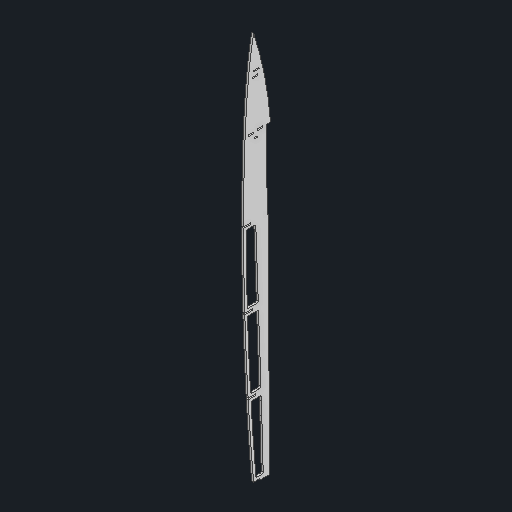
# Autodesk Inventor part: stringer
Saved by Autodesk Inventor 2023 (Build 270158030, 158C)
## iProperties
Created: 2022-03-21
Part Number: stringer
Material: Generic
Document SubType Name: Modeling
Designer: kardo
Density: 1 g/cm^3
Appearance: Default
Mass: 50.8397 g
Surface Area: 402.853 cm^2
Volume: 50.8397 cm^3
Author: kardo
Autodesk Inventor part; units mm, degrees
ref_plane "YZ Plane" through (0, 0, 0) normal (1, 0, 0) x (0, 1, 0)
ref_plane "XZ Plane" through (0, 0, 0) normal (0, 1, 0) x (-1, 0, 0)
ref_plane "XY Plane" through (0, 0, 0) normal (0, 0, 1) x (1, 0, 0)
derived "parameters_frame.ipt"
derived "surface_body.ipt"
sketch "sk_long_outer" plane through (0, 0, 0) normal (1, 0, 0) x (0, 1, 0)
  line L0 (-345, 107.6209) -> (-345, -224.5198) construction
  line L1 (255, 107.6209) -> (255, -224.5198) construction
  line L2 (-465, 54.4) -> (375, 54.4) construction
  line L3 (-483, 0) -> (357, 0) construction
  line L4 (0, 107.6209) -> (0, -224.5198) construction
  line L5 (0, 14.144) -> (-345, 11.968)
  line L6 (-345, 11.968) -> (-345, 39.712)
  line L7 (-345, 39.712) -> (0, 54.4)
  line L8 (0, 54.4) -> (255, 36.448)
  line L9 (0, 0) -> (122.4, 9.6331)
  line L10 (122.4, 9.6331) -> (255, 36.448)
  line L11 (0, 14.144) -> (0, 0)
  line L12 (0, 14.144) -> (121.9006, 15.9783)
  line L13 (121.9006, 15.9783) -> (122.4, 9.6331)
sketch "sk_rail_sponson_tunnel" plane through (81.12, 0, 0) normal (1, 0, 0) x (0, 1, 0)
  line L0 (0, 0) -> (122.4, 9.6331)
  line L1 (111.1171, 152.996) -> (142.2856, -243.0375) construction
  spline S0 degree 2 poles (122.4, 9.6331) (190.08, 14.9596) (255, 36.448) knots 0 0 0 1 1 1
sketch "sk_rail_top_tunnel" plane through (81.12, 0, 0) normal (1, 0, 0) x (0, 1, 0)
  line L0 (255, 107.6209) -> (255, -224.5198) construction
  line L1 (0, 107.6209) -> (0, -224.5198) construction
  line L2 (-345, 107.6209) -> (-345, -224.5198) construction
  line L3 (-345, 0) -> (0, 0) construction
  line L4 (-172.5, 48.8998) -> (-172.5, 0) construction
  line L5 (0, 52.89) -> (37.026, 52.89) construction
  line L6 (37.026, 52.89) -> (80.784, 47.0555) construction
  line L7 (80.784, 47.0555) -> (112.2, 37.536) construction
  line L8 (112.2, 107.6209) -> (112.2, -224.5198) construction
  line L9 (0, 52.89) -> (255, 52.89) construction
  line L10 (-469.9275, 0) -> (379.2584, 0) construction
  spline S0 degree 3 poles (0, 52.89) (92.8353, 52.89) (195.0311, 49.5089) (255, 36.448) knots 0 0 0 0 1 1 1 1
  spline S1 degree 3 poles (0, 52.89) (37.026, 52.89) (80.784, 47.0555) (112.2, 37.536) knots 1 1 1 1 2 2 2 2
  spline S2 degree 4 poles (-345, 37.3935) (-258.8686, 45.1235) (-172.5923, 49.7074) (-86.3167, 52.89) (0, 52.89) knots 0 0 0 0 0 1 1 1 1 1
  point P0 (153, 48.7795)
  point P1 (112.2, 28.832)
  point P2 (-230.0001, 45.8224)
  point P3 (-114.9999, 50.9907)
sketch "sk_rail_bottom_tunnel" plane through (81.12, 0, 0) normal (1, 0, 0) x (0, 1, 0)
  line L0 (-241.5001, 19.2432) -> (11.22, 28.376)
  arc A0 (36.465, 28.832) -> (11.22, 28.376) centre (36.465, -670.197) ccw
  line L1 (36.465, 28.832) -> (112.2, 28.832)
  arc A1 (-262.2001, 18.586) -> (-241.5001, 19.2432) centre (-326.8578, 2381.2399) ccw
  line L2 (-345, 16.32) -> (-262.2001, 18.586)
  point P0 (0, 0)
ref_plane "plane_middle" through (0, 0, 0) normal (0, 1, 0) x (-1, 0, 0)
ref_plane "plane_tunnel_right" through (81.12, 0, 0) normal (1, 0, 0) x (0, 1, 0)
ref_plane "plane_tail_1" through (0, -114.9999, 0) normal (0, 1, 0) x (-1, 0, 0)
ref_plane "plane_tail_2" through (0, -230.0001, 0) normal (0, 1, 0) x (-1, 0, 0)
derived "stencil_frame.ipt"
sketch "sk_joint_locations" plane through (81.12, 0, 0) normal (1, 0, 0) x (0, 1, 0)
  line L0 (0, 0) -> (122.4, 9.6331) construction
  line L1 (36.465, 28.832) -> (112.2, 28.832) construction
  arc A0 (36.465, 28.832) -> (11.22, 28.376) centre (36.465, -670.197) ccw construction
  line L2 (-241.5001, 19.2432) -> (11.22, 28.376) construction
  line L3 (-345, 16.32) -> (-262.2001, 18.586) construction
  arc A1 (-262.2001, 18.586) -> (-241.5001, 19.2432) centre (-326.8578, 2381.2399) ccw construction
  line L4 (-122.4795, 3121.122) -> (270.8781, -1876.9598) construction
  line L5 (-230.0001, 3089.1136) -> (-230.0001, -1866.0023) construction
  line L6 (-114.9999, 3089.1136) -> (-114.9999, -1866.0023) construction
  line L7 (-345, 3089.1136) -> (-345, -1866.0023) construction
  line L8 (0, 3089.1136) -> (0, -1866.0023) construction
  line L9 (529.622, 47.2379) -> (-602.608, 2.7525) construction
  line L10 (-673.1615, -36.5999) -> (647.9226, 67.3717) construction
  line L11 (193.439, 30.0262) -> (193.1249, 38.02) construction
  line L12 (201.1327, 36.2333) -> (201.7624, 28.2333) construction
  line L13 (0, 14.144) -> (121.9006, 15.9783) construction
  line L14 (-230.0001, 45.8224) -> (-230.0001, 19.6588) construction
  line L15 (-345, 37.3935) -> (-345, 16.32) construction
  line L16 (-114.9999, 50.9907) -> (-114.9999, 23.8147) construction
  line L17 (0, 52.89) -> (0, 27.9705) construction
  line L18 (119.1768, 50.5875) -> (119.7216, 43.6656) construction
  line L19 (120.2663, 36.7438) -> (119.7216, 43.6656) construction
  line L20 (120.2663, 36.7438) -> (120.8111, 29.822) construction
  line L21 (120.8111, 29.822) -> (121.3559, 22.9001) construction
  line L22 (121.3559, 22.9001) -> (121.9006, 15.9783) construction
  line L23 (0, 14.144) -> (0, 0) construction
  spline S0 degree 4 poles (-345, 37.3935) (-258.8686, 45.1235) (-172.5923, 49.7074) (-86.3167, 52.89) (0, 52.89) knots 0 0 0 0 0 1 1 1 1 1
  spline S1 degree 3 poles (0, 52.89) (92.8353, 52.89) (195.0311, 49.5089) (255, 36.448) knots 0 0 0 0 1 1 1 1
  spline S2 degree 2 poles (122.4, 9.6331) (190.08, 14.9596) (255, 36.448) knots 0 0 0 1 1 1
  line L24 (112.2, 37.536) -> (112.2, 28.832) construction
  line L25 (112.2, 35.548) -> (112.2, 30.82) construction
  point P0 (193.282, 34.0231)
  point P1 (201.4475, 32.2333)
  point P2 (-345, 26.8568)
  point P3 (-230.0001, 32.7406)
  point P4 (-114.9999, 37.4027)
  point P5 (0, 40.4303)
  point P6 (112.2, 33.184)
sketch "sk_stringer_base" plane through (81.12, 0, 0) normal (1, 0, 0) x (0, 1, 0)
  line L0 (0, 14.144) -> (-345, 11.968) construction
  spline S0 degree 4 poles (-345, 37.3935) (-258.8686, 45.1235) (-172.5923, 49.7074) (-86.3167, 52.89) (0, 52.89) knots 0 0 0 0 0 1 1 1 1 1 construction
  spline S1 degree 3 poles (0, 52.89) (37.026, 52.89) (80.784, 47.0555) (112.2, 37.536) knots 1 1 1 1 2 2 2 2 construction
  spline S2 degree 3 poles (0, 52.89) (92.8353, 52.89) (195.0311, 49.5089) (255, 36.448) knots 0 0 0 0 1 1 1 1 construction
  spline S3 degree 2 poles (122.4, 9.6331) (190.08, 14.9596) (255, 36.448) knots 0 0 0 1 1 1 construction
  line L1 (0, 0) -> (122.4, 9.6331) construction
  line L2 (-345, 16.32) -> (-262.2001, 18.586) construction
  arc A0 (-262.2001, 18.586) -> (-241.5001, 19.2432) centre (-326.8578, 2381.2399) ccw construction
  line L3 (-241.5001, 19.2432) -> (11.22, 28.376) construction
  arc A1 (36.465, 28.832) -> (11.22, 28.376) centre (36.465, -670.197) ccw construction
  line L4 (36.465, 28.832) -> (112.2, 28.832) construction
  line L5 (0, 2991.5273) -> (0, -1280.4843) construction
  line L6 (-345, 26.8568) -> (-345, 11.968)
  line L7 (-345, 11.968) -> (0, 14.144)
  line L8 (120.312, 10.6725) -> (119.8025, 17.1468)
  line L9 (0, 14.144) -> (0, 15.344)
  line L10 (0, 15.344) -> (119.8025, 17.1468)
  line L11 (-345, 26.8568) -> (-343, 26.8568)
  line L12 (-343, 26.8568) -> (-343, 36.3676)
  line L13 (-230.0001, 32.7406) -> (-228.0001, 32.7406)
  line L14 (-228.0001, 32.7406) -> (-228.0001, 44.7367)
  line L15 (-230.0001, 32.7406) -> (-230.0001, 44.6204)
  line L16 (-114.9999, 37.4027) -> (-114.9999, 49.7901)
  line L17 (-114.9999, 37.4027) -> (-112.9999, 37.4027)
  line L18 (-112.9999, 37.4027) -> (-112.9999, 49.8526)
  line L19 (0, 51.69) -> (0, 40.4303)
  line L20 (0, 40.4303) -> (2, 40.4303)
  line L21 (2, 40.4303) -> (2, 51.6895)
  line L22 (119.7216, 43.6656) -> (120.2663, 36.7438)
  line L23 (120.2663, 36.7438) -> (118.2725, 36.5869)
  line L24 (118.2725, 36.5869) -> (117.7277, 43.5087)
  line L25 (117.7277, 43.5087) -> (119.7216, 43.6656)
  line L26 (120.8111, 29.822) -> (118.8173, 29.665)
  line L27 (118.8173, 29.665) -> (119.362, 22.7432)
  line L28 (119.362, 22.7432) -> (121.3559, 22.9001)
  line L29 (120.8111, 29.822) -> (121.3559, 22.9001)
  line L30 (193.1249, 38.02) -> (193.439, 30.0262)
  line L31 (201.1327, 36.2333) -> (201.7624, 28.2333)
  line L32 (201.7624, 28.2333) -> (199.7685, 28.0764)
  line L33 (199.7685, 28.0764) -> (199.1389, 36.0764)
  line L34 (199.1389, 36.0764) -> (201.1327, 36.2333)
  line L35 (193.1249, 38.02) -> (191.1265, 37.9415)
  line L36 (191.1265, 37.9415) -> (191.4405, 29.9477)
  line L37 (191.4405, 29.9477) -> (193.439, 30.0262)
  line L38 (122.3058, 10.8294) -> (120.312, 10.6725)
  line L39 (110.2, 35.548) -> (112.2, 35.548)
  line L40 (112.2, 35.548) -> (112.2, 30.82)
  line L41 (112.2, 30.82) -> (110.2, 30.82)
  line L42 (110.2, 30.82) -> (110.2, 35.548)
  spline S4 degree 5 poles (-343, 36.3676) (-274.5822, 42.4668) (-206.0006, 46.7215) (-137.3775, 49.7989) (-68.6892, 51.6902) (0, 51.69) knots 0 0 0 0 0 0 1 1 1 1 1 1
  spline S5 degree 5 poles (0, 51.69) (14.1108, 51.69) (28.2217, 51.6249) (42.3321, 51.4877) (70.2924, 51.0558) (98.2445, 50.2552) (112.0882, 49.7555) (138.5614, 48.5709) (165.0044, 46.8436) (177.6143, 45.8726) (200.6905, 43.7703) (223.6773, 40.852) (234.0881, 39.3135) (244.4634, 37.5139) (254.7446, 35.2755) knots 0 0 0 0 0 0 0.275975 0.275975 0.275975 0.546891 0.546891 0.546891 0.794217 0.794217 0.794217 1 1 1 1 1 1
  spline S6 degree 4 poles (254.6229, 37.5872) (222.5063, 26.9568) (189.5513, 18.8397) (156.0318, 13.4835) (122.3058, 10.8294) knots 0 0 0 0 0 1 1 1 1 1
  point P0 (250.3665, 36.1967)
  point P1 (121.9006, 15.9783)
  dimension "d4" = 1.2
  dimension "d14" = 1.2
  dimension "d8" = 1.2
  dimension "d9" = 2
  dimension "d11" = 2
  dimension "d16" = 2
  dimension "d17" = 1.2
  constraints: 74 end point, 12 perpendicular, 7 vertical, 6 equal length, 6 parallel, 2 coincident, 2 collinear, 2 horizontal, 18 other
  measures "d8" distance of L7.end L9.end
  measures "d9" distance of L6.start L11.end
  measures "d11" distance of L19.end L20.end
  measures "d16" distance between parallel lines of L40 L42
  measures "d17" distance from line of point (121.901, 15.978) L10
extrude "thicken" add sketch "sk_stringer_base" along normal blind 3 contours L11 L12 S4 L15 L13 L14 L16 L17 L18 L19 L20 L21 S5 S6 L38 L8 L10 L9 L7 L6
sketch "sk_cut_weight" plane through (81.12, 0, 0) normal (1, 0, 0) x (0, 1, 0)
  spline S0 degree 4 poles (-345, 37.3935) (-258.8686, 45.1235) (-172.5923, 49.7074) (-86.3167, 52.89) (0, 52.89) knots 0 0 0 0 0 1 1 1 1 1 construction
  spline S1 degree 3 poles (0, 52.89) (37.026, 52.89) (80.784, 47.0555) (112.2, 37.536) knots 1 1 1 1 2 2 2 2 construction
  line L0 (36.465, 28.832) -> (112.2, 28.832) construction
  arc A0 (36.465, 28.832) -> (11.22, 28.376) centre (36.465, -670.197) ccw construction
  line L1 (-241.5001, 19.2432) -> (11.22, 28.376) construction
  arc A1 (-262.2001, 18.586) -> (-241.5001, 19.2432) centre (-326.8578, 2381.2399) ccw construction
  line L2 (-345, 16.32) -> (-262.2001, 18.586) construction
  line L3 (112.2, 37.536) -> (112.2, 28.832) construction
  line L4 (105.6257, 34.032) -> (36.465, 34.032)
  arc A2 (36.465, 34.032) -> (11.0322, 33.5726) centre (36.465, -670.197) ccw
  line L5 (11.0322, 33.5726) -> (-241.6879, 24.4398)
  arc A3 (-262.3423, 23.784) -> (-241.6879, 24.4398) centre (-326.8578, 2381.2399) ccw
  line L6 (-262.3423, 23.784) -> (-339, 21.6861)
  line L7 (-345, 16.32) -> (-345, 37.3935) construction
  line L8 (-343, 46.2922) -> (-343, 7.6751) construction
  line L9 (-228.0001, 59.5201) -> (-228.0001, 2.898) construction
  line L10 (-112.9999, 68.9991) -> (-112.9999, 15.2181) construction
  line L11 (0, 2991.5273) -> (0, -1280.4843) construction
  line L12 (-230.0001, 2991.5273) -> (-230.0001, -1280.4843) construction
  line L13 (-114.9999, 2991.5273) -> (-114.9999, -1280.4843) construction
  line L14 (-339, 21.6861) -> (-339, 32.7062)
  line L15 (-234.0001, 40.3779) -> (-234.0001, 24.7176)
  line L16 (-224.0001, 40.9599) -> (-224.0001, 25.079)
  line L17 (-118.9999, 45.66) -> (-118.9999, 28.8735)
  line L18 (-108.9999, 45.973) -> (-108.9999, 29.2349)
  line L19 (-4, 47.6874) -> (-4, 33.0294)
  spline S2 degree 5 poles (-339, 32.7062) (-271.3751, 38.6568) (-203.5939, 42.8243) (-135.7716, 45.8406) (-67.8862, 47.6901) (0, 47.69) knots 0 0 0 0 0 0 1 1 1 1 1 1
  spline S3 degree 5 poles (0, 47.69) (7.6283, 47.6899) (15.2566, 47.4808) (22.8775, 47.097) (38.2152, 45.9964) (53.4935, 44.2547) (61.1715, 43.2182) (74.7402, 41.0892) (88.2037, 38.3793) (94.0473, 37.0771) (99.8603, 35.6399) (105.6257, 34.032) knots 0 0 0 0 0 0 0.357145 0.357145 0.357145 0.719774 0.719774 0.719774 1 1 1 1 1 1
  point P0 (0, 0)
  dimension "d20" = 5.2
  dimension "d21" = 2
  dimension "d22" = 2
  dimension "d23" = 2
  dimension "d25" = 4
  dimension "d26" = 4
  dimension "d27" = 4
  dimension "d28" = 4
  dimension "d29" = 4
  dimension "d30" = 4
  constraints: 29 end point, 10 parallel, 5 point on line, 4 point on circle, 2 centre point, 16 other
  measures "d21" distance between parallel lines of L7 L8
  measures "d22" distance between parallel lines of L12 L9
  measures "d23" distance between parallel lines of L13 L10
  measures "d25" distance between parallel lines of L8 L14
  measures "d26" distance between parallel lines of L12 L15
  measures "d27" distance between parallel lines of L9 L16
  measures "d28" distance between parallel lines of L17 L13
  measures "d29" distance between parallel lines of L18 L10
  measures "d30" distance between parallel lines of L19 L11
extrude "cut_weight" cut sketch "sk_cut_weight" along normal through all both and the other way through all contours L19 L5 L18 S2 | L17 L5 L16 S2 | L15 L5 A3 L6 L14 S2
fillet "rounding" radius 2 12 edges at (82.62, -4, 33.0294) (82.62, -4, 47.6874) (82.62, -118.9999, 45.66) (82.62, -234.0001, 40.3779) (82.62, -234.0001, 24.7176) (82.62, -118.9999, 28.8735) (82.62, -339, 21.6861) (82.62, -224.0001, 25.079) (82.62, -108.9999, 29.2349) (82.62, -108.9999, 45.973) (82.62, -224.0001, 40.9599) (82.62, -339, 32.7062)
equation "\"d4\" = shell_thickness"
equation "\"d14\" = shell_thickness"
equation "\"d8\" = shell_thickness"
equation "\"d9\" = bulkhead_thickness"
equation "\"d11\" = bulkhead_thickness"
equation "\"d16\" = bulkhead_thickness"
equation "\"d17\" = shell_thickness"
equation "\"d12\" = stringer_thickness"
equation "\"d20\" = bulkhead_inset + shell_thickness"
equation "\"d21\" = bulkhead_thickness"
equation "\"d22\" = bulkhead_thickness"
equation "\"d23\" = bulkhead_thickness"
equation "\"d25\" = bulkhead_inset"
equation "\"d26\" = bulkhead_inset"
equation "\"d27\" = bulkhead_inset"
equation "\"d28\" = bulkhead_inset"
equation "\"d29\" = bulkhead_inset"
equation "\"d30\" = bulkhead_inset"
equation "\"d34\" = 0.5 * bulkhead_inset"
equation "\"shell_thickness\" = 1.2"
equation "\"bulkhead_thickness\" = 2"
equation "\"stringer_thickness\" = 3"
equation "\"bulkhead_inset\" = 4"
body "Solid1"
